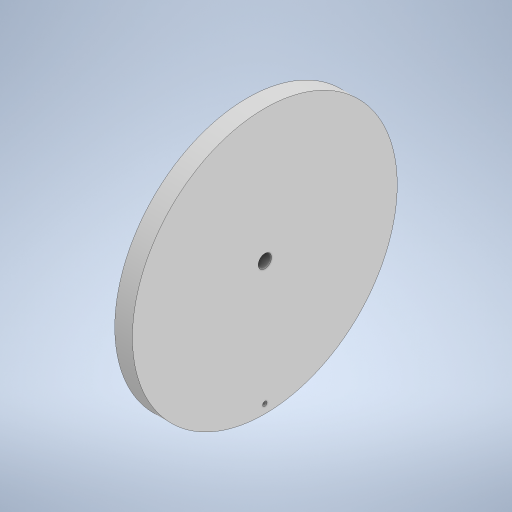
# Autodesk Inventor part: Langbektang houder
Saved by Autodesk Inventor 2023.2 (Build 272271000, 271)
## iProperties
Created: 2020-09-09
Part Number: Langbektang houder
Material: Generic
Document SubType Name: Modeling
Designer: nathan.bollaert
Density: 1 g/cm^3
Appearance: Default
Author: nathan.bollaert
Autodesk Inventor part; units mm, degrees
ref_plane "YZ Plane" through (0, 0, 0) normal (1, 0, 0) x (0, 1, 0)
ref_plane "XZ Plane" through (0, 0, 0) normal (0, 1, 0) x (-1, 0, 0)
ref_plane "XY Plane" through (0, 0, 0) normal (0, 0, 1) x (1, 0, 0)
sketch "Sketch1" plane through (0, 0, 0) normal (1, 0, 0) x (0, 1, 0)
  circle A0 centre (0, 0) radius 30
  dimension "d228" = 60
  constraints: 1 centre point, 1 coincident
  measures "d228" diameter of A0
extrude "Extrusion1" add sketch "Sketch1" along normal blind 4
hole "Hole1" at (0, 0, 0) direction (1, 0, 0) diameter 3 end through all
sketch "Sketch2" plane through (4, 0, 0) normal (1, 0, 0) x (0, 0, -1)
  circle A0 centre (0, -28) radius 0.5
  circle A1 centre (0, 0) radius 30 projected
  dimension "d238" = 1
  dimension "d239" = 28
  constraints: 1 centre point, 1 vertical alignment
  measures "d238" diameter of A0
  measures "d239" distance of A1.centre A0.centre
hole "Hole2" at (4, -28, 0) direction (-1, 0, 0) diameter 1 end through all
body "Solid5"
